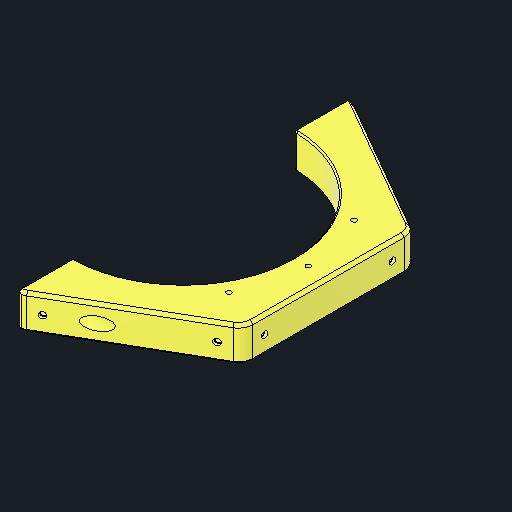
# Autodesk Inventor part: Baseplate-for-ICF152-flange-outer-part
Saved by Autodesk Inventor 2026 (Build 300175050, 175E)
## iProperties
Created: 2023-12-01
Part Number: Baseplate-for-ICF152-flange-outer-part
Material: Generic
Document SubType Name: Modeling
Designer: kuzmin
Density: 1 g/cm^3
Appearance: Smooth - Yellow
Author: kuzmin
Autodesk Inventor part; units mm, degrees
note: some values were not read from the file. Chosen so that the rebuilt part matches the saved one: direction of "Hole2"; pattern direction of "Circular Pattern1".
ref_plane "YZ Plane" through (0, 0, 0) normal (1, 0, 0) x (0, 1, 0)
ref_plane "XY Plane" through (0, 0, 0) normal (0, 0, 1) x (1, 0, 0)
sketch "Sketch1" plane through (0, 0, 0) normal (0, 0, 1) x (1, 0, 0)
  circle A0 centre (0, 0) radius 76
  line L0 (57.735, -100) -> (-57.735, -100)
  line L1 (-57.735, -100) -> (-115.4701, 0)
  line L2 (-115.4701, 0) -> (-57.735, 100)
  line L3 (-57.735, 100) -> (57.735, 100)
  line L4 (57.735, 100) -> (115.4701, 0)
  line L5 (115.4701, 0) -> (57.735, -100)
  dimension "d0" = 152
  dimension "d1" = 200
  constraints: 12 end point, 2 coincident, 1 centre point, 1 horizontal, 13 other
  measures "d0" diameter of A0
  measures "d1" vertical distance of L0.start L2.end
extrude "Extrusion1" add sketch "Sketch1" along normal blind 24
fillet "Fillet1" radius 10 6 edges at (-57.735, 100, 12) (57.735, 100, 12) (115.4701, 0, 12) (57.735, -100, 12) (-57.735, -100, 12) (-115.4701, 0, 12)
ref_plane "Work Plane1" through (0, 0.2, 0) normal (0, 1, 0) x (-1, 0, 0)
chamfer "Chamfer2" distance 2 angle 45 24 edges at (0, -100, 24) (56.9615, -98.6603, 24) (86.6025, -50, 24) (113.923, 0, 24) (86.6025, 50, 24) (56.9615, 98.6603, 24) (0, 100, 24) (-56.9615, 98.6603, 24) (-86.6025, 50, 24) (-113.923, 0, 24) (-86.6025, -50, 24) (-56.9615, -98.6603, 24) (-86.6025, -50, 0) (-56.9615, -98.6603, 0) (0, -100, 0) (56.9615, -98.6603, 0) (86.6025, -50, 0) (113.923, 0, 0) (86.6025, 50, 0) (56.9615, 98.6603, 0) (0, 100, 0) (-56.9615, 98.6603, 0) (-86.6025, 50, 0) (-113.923, 0, 0)
split "Split1" plane through (0, 0.2, 0) removes the side toward (0, -1, 0)
fillet "Fillet3" radius 2 4 edges at (75.9997, 0.2, 12) (-75.9997, 0.2, 12) (113.921, 0.2, 12) (-113.921, 0.2, 12)
sketch "Sketch12" plane through (0, 0, 24) normal (0, 0, 1) x (1, 0, 0)
  circle A0 centre (0, 86) radius 1.7
  arc A1 (75.9698, 2.1436) -> (-75.9698, 2.1436) centre (0, 0) ccw projected
  point P0 (0, 76)
  dimension "d66" = 3.4
  dimension "d67" = 10
  constraints: 1 centre point, 1 point on circle
  measures "d66" diameter of A0
  measures "d67" distance of A0.centre point (0, 76)
extrude "Extrusion10" cut sketch "Sketch12" against normal through all
ref_plane "Work Plane3" through (0, 80.2, 0) normal (0, 1, 0) x (-1, 0, 0)
sketch "Sketch6" plane through (0, 80.2, 0) normal (0, 1, 0) x (-1, 0, 0)
  line L0 (111.6146, 0) -> (111.6146, 24) projected
  line L1 (77.969, 0) -> (111.6146, 0) projected
  line L2 (77.969, 24) -> (77.969, 0) projected
  line L3 (111.6146, 24) -> (77.969, 24) projected
  line L4 (-51.9615, 0) -> (51.9615, 0) projected
  point P0 (0, 0)
  point P1 (94.7918, 12)
  point P2 (111.6146, 12)
  point P3 (94.7918, 24)
  point P4 (0, 0)
  dimension "d73" = 94.7918
  constraints: 3 midpoint, 1 horizontal alignment, 1 vertical alignment
  measures "d73" horizontal distance of point (94.792, 12) point (0, 0)
hole "Hole2" at (-94.7918, 80.2, 12) direction (0, -1, 0) diameter 4.5 depth 80 counterbore diameter 9 counterbore depth 70
sketch "Sketch7" plane through (-111.6146, 0.2, 0) normal (0, -1, 0) x (1, 0, 0)
  circle A0 centre (16.8228, 12) radius 2.25 projected
  circle A1 centre (16.8228, 12) radius 2.8
  point P0 (111.6146, 0)
  dimension "d42" = 5.6
  constraints: 1 centre point, 1 coincident
  measures "d42" diameter of A1
extrude "Extrusion5" cut sketch "Sketch7" against normal blind 2.5
mirror "Mirror2" about plane through (0, 0, 0) normal (1, 0, 0) of "Extrusion5", "Hole2"
chamfer "Chamfer4" distance 1 angle 45 14 edges at (0, 76, 0) (-76.5748, 0.766, 0) (76.5748, 0.766, 0) (94.7918, 0.2, 0) (111.7677, 0.2059, 0) (-94.7918, 0.2, 0) (-111.7677, 0.2059, 0) (0, 76, 24) (-76.5748, 0.766, 24) (76.5748, 0.766, 24) (94.7918, 0.2, 24) (111.7677, 0.2059, 24) (-94.7918, 0.2, 24) (-111.7677, 0.2059, 24)
sketch "Sketch8" plane through (60.6218, 95, 22) normal (0.8660254, 0.5, 0) x (0, 0, -1)
  circle A0 centre (10, -8) radius 1.75
  circle A1 centre (10, -95.923) radius 1.75
  ellipse E0 centre (10, -68.34) end of major axis (10, -77.34) minor radius 4.5 projected
  line L0 (20, 0) -> (20, -103.923) projected
  line L1 (0, 0) -> (20, 0) projected
  line L2 (0, -103.923) -> (0, 0) projected
  line L3 (20, -103.923) -> (0, -103.923) projected
  point P0 (22, -51.9615)
  point P1 (10, 0)
  dimension "d48" = 3.5
  dimension "d49" = 8
  dimension "d65" = 8
  constraints: 2 centre point, 2 vertical alignment, 1 equal radius, 1 midpoint, 1 other
  measures "d48" diameter of A1
  measures "d49" distance from line of L3 A1.centre
  measures "d65" distance from line of L1 A0.centre
extrude "Extrusion6" cut sketch "Sketch8" against normal blind 10 contours A0 | A1
sketch "Sketch9" plane through (60.6218, 95, 22) normal (0.8660254, 0.5, 0) x (0, 0, -1)
  circle A0 centre (10, -95.923) radius 1.75 projected
  circle A1 centre (10, -8) radius 1.75 projected
  circle A2 centre (10, -95.923) radius 1.75 projected
  circle A3 centre (10, -95.923) radius 2.25
  circle A4 centre (10, -8) radius 1.75 projected
  circle A5 centre (10, -8) radius 2.25
  point P0 (22, -51.9615)
  dimension "d54" = 4.5
  constraints: 2 centre point, 2 coincident, 1 equal radius
  measures "d54" diameter of A3
extrude "Extrusion7" cut sketch "Sketch9" against normal blind 2 contours A1 | A3 | A5
mirror "Mirror3" about plane through (0, 0, 0) normal (1, 0, 0) of "Extrusion6", "Extrusion7"
sketch "Sketch10" plane through (-51.9615, 100, 2) normal (0, 1, 0) x (1, 0, 0)
  circle A0 centre (95.923, -10) radius 1.7
  circle A1 centre (8, -10) radius 1.7
  line L0 (103.923, 0) -> (103.923, -20) projected
  line L1 (0, -20) -> (0, 0) projected
  point P0 (51.9615, 2)
  point P1 (103.923, -10)
  dimension "d57" = 8
  dimension "d58" = 8
  dimension "d59" = 3.4
  constraints: 2 centre point, 2 horizontal alignment, 1 equal radius, 1 midpoint
  measures "d57" distance from line of L0 A0.centre
  measures "d58" distance from line of L1 A1.centre
  measures "d59" diameter of A0
extrude "Extrusion8" cut sketch "Sketch10" against normal blind 10
sketch "Sketch11" plane through (-51.9615, 100, 2) normal (0, 1, 0) x (1, 0, 0)
  circle A0 centre (95.923, -10) radius 1.7 projected
  circle A1 centre (95.923, -10) radius 2.2
  circle A2 centre (8, -10) radius 1.7 projected
  circle A3 centre (8, -10) radius 2.2
  point P0 (51.9615, 2)
  dimension "d62" = 4.4
  constraints: 2 centre point, 2 coincident, 1 equal radius
  measures "d62" diameter of A3
extrude "Extrusion9" cut sketch "Sketch11" against normal blind 2 contours A0 | A1 | A2 | A3
pattern_circular "Circular Pattern1" count 3 over 60 about axis through (0, 0, 0) along (0, 0, 1) of "Extrusion10" both ways yes
body "Solid1"
